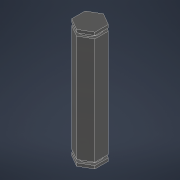
# Autodesk Inventor part: Wasp Intermediate Axel
Saved by Autodesk Inventor 2022 (Build 260153000, 153)
## iProperties
Created: 2022-09-18
Part Number: Wasp Intermediate Axel
Material: Generic
Document SubType Name: Modeling
Designer: robpl
Density: 1 g/cm^3
Appearance: Dark Gray
Author: robpl
Autodesk Inventor part; units mm, degrees
ref_plane "YZ Plane" through (0, 0, 0) normal (1, 0, 0) x (0, 1, 0)
ref_plane "XZ Plane" through (0, 0, 0) normal (0, 1, 0) x (-1, 0, 0)
ref_plane "XY Plane" through (0, 0, 0) normal (0, 0, 1) x (1, 0, 0)
sketch "Sketch1" plane through (0, 0, 0) normal (0, 1, 0) x (-1, 0, 0)
  line L0 (4.7625, 2.7496) -> (4.7625, -2.7496)
  line L1 (4.7625, -2.7496) -> (0, -5.4993)
  line L2 (0, -5.4993) -> (-4.7625, -2.7496)
  line L3 (-4.7625, -2.7496) -> (-4.7625, 2.7496)
  line L4 (-4.7625, 2.7496) -> (0, 5.4993)
  line L5 (0, 5.4993) -> (4.7625, 2.7496)
  point P0 (0, 0)
  point P1 (0, 0)
  dimension "d0" = 9.525
  constraints: 12 end point, 1 coincident, 1 vertical, 13 other
  measures "d0" distance between parallel lines of L3 L0
extrude "Extrusion1" add sketch "Sketch1" along normal blind 49.8
sketch "Sketch2" plane through (0, 0, 0) normal (1, 0, 0) x (0, 1, 0)
  line L0 (1.2, 14) -> (2.4, 14)
  line L1 (2.4, 14) -> (2.4, 4)
  line L2 (2.4, 4) -> (1.2, 4)
  line L3 (1.2, 4) -> (1.2, 14)
  line L4 (0, -2.7496) -> (0, 2.7496) projected
  line L5 (-9.48, 0) -> (56.88, 0) projected
  line L6 (47.4, 14) -> (46.2, 14)
  line L7 (46.2, 14) -> (46.2, 4)
  line L8 (46.2, 4) -> (47.4, 4)
  line L9 (47.4, 4) -> (47.4, 14)
  point P0 (0, 0)
  point P1 (0, 0)
  point P2 (1.8, 14)
  dimension "d3" = 1.2
  dimension "d4" = 1.2
  dimension "d5" = 4
  dimension "d6" = 10
  dimension "d8" = 43.8
  constraints: 16 end point, 4 parallel, 2 equal length, 2 horizontal, 2 perpendicular, 1 coincident, 1 horizontal alignment, 1 midpoint
  measures "d3" distance of L0.start L0.end
  measures "d4" distance between parallel lines of L4 L3
  measures "d5" vertical distance of L2.end point (0, 0)
  measures "d6" distance of L2.end L0.start
  measures "d8" distance between parallel lines of L7 L1
revolve "Revolution1" cut sketch "Sketch2" angle 360 about axis through (0, -10, 0) along (0, 1, 0)
sketch "Sketch3" plane through (0, 49.8, 0) normal (0, 1, 0) x (1, 0, 0)
  line L0 (0, -5.4993) -> (4.7625, -2.7496) projected
  line L1 (4.7625, -2.7496) -> (4.7625, 2.7496) projected
  line L2 (4.7625, 2.7496) -> (0, 5.4993) projected
  line L3 (0, 5.4993) -> (-4.7625, 2.7496) projected
  line L4 (-4.7625, 2.7496) -> (-4.7625, -2.7496) projected
  line L5 (-4.7625, -2.7496) -> (0, -5.4993) projected
  point P0 (0, 0)
extrude "Extrusion2" cut sketch "Sketch3" against normal blind 1.2
body "Solid1"
